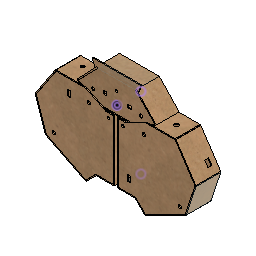
Ivrida_Digimod (Autodesk Fusion 360 design; units mm, degrees)
Autodesk Fusion 360 part; units mm, degrees
sketch "Sketch1" plane through (0, 0, 0) normal (0, 1, 0) x (1, 0, 0) in component "DigiMod"
  line L0 (0, 0) -> (120, 0)
  line L1 (120, 0) -> (160, 60)
  line L2 (160, 60) -> (140, 120)
  line L3 (140, 120) -> (60, 160)
  line L4 (60, 160) -> (40, 140)
  line L5 (40, 140) -> (-40, 140)
  line L6 (-40, 140) -> (-60, 160)
  line L7 (-60, 160) -> (-140, 120)
  line L8 (-140, 120) -> (-160, 60)
  line L9 (-160, 60) -> (-120, 0)
  line L10 (-120, 0) -> (0, 0)
  constraint coincident L0.start L10.end
  constraint horizontal L0
  constraint horizontal L5
  constraint perpendicular L4 L6
  constraint parallel L0 L10
extrude "Extrude1" add sketch "Sketch1" along normal blind 50 makes body 1 in component "DigiMod"
sketch "Sketch2" plane through (0, 0, 0) normal (0, 1, 0) x (1, 0, 0) in component "DigiMod"
  line L0 (0, 0) -> (3, 0)
  line L1 (3, 0) -> (3, 105.3915)
  line L2 (3, 105.3915) -> (3, 140)
  line L3 (3, 140) -> (-3, 140)
  line L4 (-3, 140) -> (-3, 0)
  line L5 (-3, 0) -> (0, 0)
  constraint coincident L0.start L5.end
  constraint horizontal L0
  constraint perpendicular L0 L1
  constraint perpendicular L0 L2
  constraint perpendicular L2 L3
  constraint perpendicular L3 L4
  constraint perpendicular L4 L5
extrude "Extrude2" cut sketch "Sketch2" along normal blind 48 bodies 1 in component "DigiMod"
extrude "Extrude3" add 1 faces at (27.6667, 32.6667, -140) along direction (0, 0, -1) blind 2 on bodies 1 bodies 1 in component "DigiMod"
extrude "Extrude4" cut 1 faces at (-46.6667, 16.6667, -146.6667) along direction (0.707107, 0, -0.707107) blind 2 on bodies 1 bodies 1 in component "DigiMod"
extrude "Extrude5" add 1 faces at (-86.6667, 33.3333, -146.6667) along direction (-0.447214, 0, -0.894427) blind 2 on bodies 1 bodies 1 in component "DigiMod"
extrude "Extrude6" add 1 faces at (-46.6667, 16.6667, -146.6667) along direction (0.707107, 0, -0.707107) blind 2 on bodies 1 bodies 1 in component "DigiMod"
extrude "Extrude7" add 1 faces at (-146.6667, 16.6667, -100) along direction (-0.948683, 0, -0.316228) blind 2 on bodies 1 bodies 1 in component "DigiMod"
extrude "Extrude8" add 1 faces at (-146.6667, 33.3333, -40) along direction (-0.83205, 0, 0.5547) blind 2 on bodies 1 bodies 1 in component "DigiMod"
extrude "Extrude9" add 1 faces at (-81, 32.6667, 0) along direction (0, 0, 1) blind 2 on bodies 1 bodies 1 in component "DigiMod"
extrude "Extrude10" add 1 faces at (133.3333, 33.3333, -20) along direction (0.83205, 0, 0.5547) blind 2 on bodies 1 bodies 1 in component "DigiMod"
extrude "Extrude11" add 1 faces at (153.3333, 16.6667, -80) along direction (0.948683, 0, -0.316228) blind 2 on bodies 1 bodies 1 in component "DigiMod"
extrude "Extrude12" add 1 faces at (113.3333, 16.6667, -133.3333) along direction (0.447214, 0, -0.894427) blind 2 on bodies 1 bodies 1 in component "DigiMod"
extrude "Extrude13" cut 1 faces at (53.3333, 16.6667, -153.3333) along direction (-0.707107, 0, -0.707107) blind 2 on bodies 1 bodies 1 in component "DigiMod"
extrude "Extrude14" add 1 faces at (53.3333, 16.6667, -153.3333) along direction (-0.707107, 0, -0.707107) blind 2 on bodies 1 bodies 1 in component "DigiMod"
sketch "Sketch1 (2)" plane through (0, 0, 0) normal (0, -1, 0) x (1, 0, 0)
  line L0 (-39.1716, -142) -> (-3, -142)
  line L1 (-3, -142) -> (-3, 2)
  line L2 (-3, 2) -> (-120, 2)
  line L3 (-120, 2) -> (-120, 0)
  line L4 (-120, 0) -> (-121.6641, 1.1094)
  line L5 (-121.6641, 1.1094) -> (-161.6641, -58.8906)
  line L6 (-161.6641, -58.8906) -> (-160, -60)
  line L7 (-160, -60) -> (-161.8974, -60.6325)
  line L8 (-161.8974, -60.6325) -> (-141.8974, -120.6325)
  line L9 (-141.8974, -120.6325) -> (-140, -120)
  line L10 (-140, -120) -> (-140.8944, -121.7889)
  line L11 (-140.8944, -121.7889) -> (-60.8944, -161.7889)
  line L12 (-60.8944, -161.7889) -> (-60, -160)
  line L13 (-60, -160) -> (-58.5858, -161.4142)
  line L14 (-58.5858, -161.4142) -> (-39.1716, -142)
  line L15 (-5, -140) -> (-40, -140)
  line L16 (-40, -140) -> (-60, -160)
  line L17 (-60, -160) -> (-140, -120)
  line L18 (-140, -120) -> (-160, -60)
  line L19 (-160, -60) -> (-120, 0)
  line L20 (-120, 0) -> (-75, 0)
  line L21 (-5, -140) -> (-5, -20)
  line L22 (-5, -20) -> (-40, -20)
  line L23 (-40, -20) -> (-75, 0)
  constraint perpendicular L1 L15
  constraint coincident L12.end L13.start
  constraint coincident L9.end L10.start
  constraint coincident L6.end L7.start
  constraint coincident L3.end L4.start
  constraint perpendicular L3 L20
  constraint perpendicular L15 L21
  constraint perpendicular L1 L22
extrude "Extrude15" cut sketch "Sketch1 (2)" against normal blind 48 contours L15 L16 L17 L18 L19 L20 L21 L22 L23 bodies 1 in component "DigiMod"
sketch "Sketch2 (2)" plane through (0, 0, 0) normal (0, -1, 0) x (1, 0, 0)
  line L0 (60, -160) -> (60.8944, -161.7889)
  line L1 (60.8944, -161.7889) -> (140.8944, -121.7889)
  line L2 (140.8944, -121.7889) -> (140, -120)
  line L3 (140, -120) -> (141.8974, -120.6325)
  line L4 (141.8974, -120.6325) -> (161.8974, -60.6325)
  line L5 (161.8974, -60.6325) -> (160, -60)
  line L6 (160, -60) -> (161.6641, -58.8906)
  line L7 (161.6641, -58.8906) -> (121.6641, 1.1094)
  line L8 (121.6641, 1.1094) -> (120, 0)
  line L9 (120, 0) -> (120, 2)
  line L10 (120, 2) -> (3, 2)
  line L11 (3, 2) -> (3, -142)
  line L12 (3, -142) -> (39.1716, -142)
  line L13 (39.1716, -142) -> (58.5858, -161.4142)
  line L14 (58.5858, -161.4142) -> (60, -160)
  line L15 (40, -140) -> (5, -140)
  line L16 (5, -140) -> (5, -20)
  line L17 (5, -20) -> (40, -20)
  line L18 (40, -20) -> (75, 0)
  line L19 (75, 0) -> (120, 0)
  line L20 (120, 0) -> (160, -60)
  line L21 (160, -60) -> (140, -120)
  line L22 (140, -120) -> (60, -160)
  line L23 (40, -140) -> (60, -160)
  constraint perpendicular L11 L15
  constraint perpendicular L15 L16
  constraint perpendicular L16 L17
  constraint coincident L8.end L9.start
  constraint perpendicular L9 L19
  constraint coincident L5.end L6.start
  constraint coincident L2.end L3.start
  constraint coincident L0.start L14.end
  constraint perpendicular L14 L23
extrude "Extrude16" cut sketch "Sketch2 (2)" against normal blind 48 contours L15 L16 L17 L18 L19 L20 L21 L22 L23 bodies 1 in component "DigiMod"
sketch "Sketch3" plane through (0, 0, 2) normal (0, 0, 1) x (-1, 0, 0)
  line L0 (3, 0) -> (3, -48)
  line L1 (3, -48) -> (-3, -48)
  line L2 (-3, 0) -> (-120, 0)
  line L3 (-120, 0) -> (-120, -50)
  line L4 (-120, -50) -> (120, -50)
  line L5 (120, -50) -> (120, 0)
  line L6 (120, 0) -> (3, 0)
sketch "Sketch4" plane through (0, 0, 2) normal (0, 0, 1) x (-1, 0, 0)
sketch "Sketch5" plane through (0, 0, 2) normal (0, 0, 1) x (1, 0, 0)
  line L0 (-3, 48) -> (-40, 48)
  line L1 (-40, 48) -> (-40, 0)
  line L2 (-40, 0) -> (-3, 0)
  line L3 (-3, 0) -> (-3, 48)
  point P0 (-3, 48)
  point P1 (-40, 48)
  point P2 (-40, 0)
  point P3 (-3, 0)
  constraint coincident P0 L0.start
  constraint coincident P1 L0.end
  constraint coincident P2 L1.end
  constraint coincident P3 L2.end
extrude "Extrude17" cut sketch "Sketch5" against normal blind 20 bodies 1 in component "DigiMod"
sketch "Sketch6" plane through (0, 48, 0) normal (0, -1, 0) x (1, 0, 0)
  line L0 (-3, -18) -> (-3, -142)
  line L1 (-3, -142) -> (3, -142)
  line L2 (3, 2) -> (-40, 2)
  line L3 (-40, 2) -> (-40, -18)
  line L4 (-40, -18) -> (-3, -18)
sketch "Sketch7" plane through (0, 0, 0) normal (0, -1, 0) x (1, 0, 0)
  line L0 (-3, -18) -> (-40, -18)
  line L1 (-40, -18) -> (-40, 2)
  line L2 (-40, 2) -> (-120, 2)
  line L3 (-120, 2) -> (-120, 0)
  line L4 (-120, 0) -> (-75, 0)
  line L5 (-75, 0) -> (-40, -20)
  line L6 (-40, -20) -> (-5, -20)
  line L7 (-5, -20) -> (-5, -140)
  line L8 (-5, -140) -> (-40, -140)
  line L9 (-40, -140) -> (-60, -160)
  line L10 (-60, -160) -> (-58.5858, -161.4142)
  line L11 (-58.5858, -161.4142) -> (-39.1716, -142)
  line L12 (-39.1716, -142) -> (-3, -142)
  line L13 (-3, -142) -> (-3, -18)
  line L14 (-40, 2) -> (-75, 2)
  line L15 (-75, 2) -> (-40, -18)
  constraint coincident L1.end L2.start
  constraint coincident L2 L14.end
  constraint perpendicular L1 L14
  constraint coincident L0.end L1.start
extrude "Extrude18" cut sketch "Sketch7" against normal blind 48 contours L1 L2 L14 L15 bodies 1 in component "DigiMod"
sketch "Sketch8" plane through (0, 0, 2) normal (0, 0, 1) x (-1, 0, 0)
sketch "Sketch9" plane through (0, 0, 2) normal (0, 0, 1) x (-1, 0, 0)
  point P0 (-3, 0)
sketch "Sketch10" plane through (0, 0, 2) normal (0, 0, 1) x (-1, 0, 0)
  line L0 (-3, -48) -> (-40, -48)
  line L1 (-40, -48) -> (-40, 0)
  line L2 (-40, 0) -> (-3, 0)
  line L3 (-3, 0) -> (-3, -48)
  point P0 (-3, -48)
  point P1 (-40, -48)
  point P2 (-40, 0)
  point P3 (-3, 0)
  constraint coincident P0 L0.start
  constraint coincident P1 L0.end
  constraint coincident P2 L1.end
  constraint coincident P3 L2.end
extrude "Extrude19" cut sketch "Sketch10" against normal blind 20 bodies 1 in component "DigiMod"
sketch "Sketch11" plane through (0, 0, 0) normal (0, -1, 0) x (1, 0, 0)
  line L0 (40, -18) -> (3, -18)
  line L1 (3, -18) -> (3, -142)
  line L2 (3, -142) -> (39.1716, -142)
  line L3 (39.1716, -142) -> (58.5858, -161.4142)
  line L4 (58.5858, -161.4142) -> (60, -160)
  line L5 (60, -160) -> (40, -140)
  line L6 (40, -140) -> (5, -140)
  line L7 (5, -140) -> (5, -20)
  line L8 (5, -20) -> (40, -20)
  line L9 (40, -20) -> (75, 0)
  line L10 (75, 0) -> (120, 0)
  line L11 (120, 0) -> (120, 2)
  line L12 (120, 2) -> (40, 2)
  line L13 (40, 2) -> (40, -18)
  line L14 (40, -18) -> (75, 2)
  line L15 (75, 2) -> (40, 2)
  constraint coincident L0.start L13.end
  constraint coincident L12 L14.end
  constraint coincident L12.end L13.start
extrude "Extrude20" cut sketch "Sketch11" against normal blind 48 contours L12 L13 L14 L15 bodies 1 in component "DigiMod"
delete_face "DeleteFace1" 1 faces at (15.3333, 48, -4.6667) on bodies 1 in component "DigiMod"
sketch "Sketch12" plane through (0, 48, 0) normal (0, -1, 0) x (1, 0, 0)
  line L0 (-5, -140) -> (-5, -20)
  line L1 (-5, -20) -> (-40, -20)
  line L2 (-40, -20) -> (-75, 0)
  line L3 (-75, 0) -> (-120, 0)
  line L4 (-120, 0) -> (-160, -60)
  line L5 (-160, -60) -> (-140, -120)
  line L6 (-140, -120) -> (-60, -160)
  line L7 (-60, -160) -> (-40, -140)
  line L8 (-40, -140) -> (-5, -140)
  line L9 (-120, 0) -> (-115, 0)
  line L10 (-115, 0) -> (-123.3146, -4.9719)
  constraint coincident L3.end L4.start
  constraint coincident L3 L9.end
  constraint parallel L3 L9
  constraint coincident L4 L10.end
extrude "Extrude1'" add sketch "Sketch12" along normal blind 46 separate body contours L3 L4 L9 L10 makes body 2
sketch "Sketch13" plane through (0, 48, 0) normal (0, -1, 0) x (1, 0, 0)
  line L0 (-5, -140) -> (-5, -20)
  line L1 (-5, -20) -> (-40, -20)
  line L2 (-40, -20) -> (-75, 0)
  line L3 (-75, 0) -> (-120, 0)
  line L4 (-120, 0) -> (-160, -60)
  line L5 (-160, -60) -> (-140, -120)
  line L6 (-140, -120) -> (-60, -160)
  line L7 (-60, -160) -> (-40, -140)
  line L8 (-40, -140) -> (-5, -140)
  line L9 (-75, 0) -> (-80, 0)
  line L10 (-80, 0) -> (-69.9937, -2.8607)
  constraint coincident L2.end L3.start
  constraint coincident L3 L9.end
  constraint parallel L3 L9
  constraint coincident L2 L10.end
extrude "Extrude2'" add sketch "Sketch13" along normal blind 46 separate body contours L2 L3 L9 L10 makes body 3
sketch "Sketch14" plane through (0, 48, 0) normal (0, -1, 0) x (1, 0, 0)
  line L0 (-5, -140) -> (-5, -20)
  line L1 (-5, -20) -> (-40, -20)
  line L2 (-40, -20) -> (-75, 0)
  line L3 (-75, 0) -> (-120, 0)
  line L4 (-120, 0) -> (-160, -60)
  line L5 (-160, -60) -> (-140, -120)
  line L6 (-140, -120) -> (-60, -160)
  line L7 (-60, -160) -> (-40, -140)
  line L8 (-40, -140) -> (-5, -140)
  line L9 (-5, -135) -> (-10, -140)
  constraint coincident L0 L9.start
  constraint coincident L8 L9.end
extrude "Extrude3'" add sketch "Sketch14" along normal blind 46 separate body contours L0 L8 L9 makes body 4
sketch "Sketch15" plane through (0, 48, 0) normal (0, -1, 0) x (1, 0, 0)
  line L0 (-5, -140) -> (-5, -20)
  line L1 (-5, -20) -> (-40, -20)
  line L2 (-40, -20) -> (-75, 0)
  line L3 (-75, 0) -> (-120, 0)
  line L4 (-120, 0) -> (-160, -60)
  line L5 (-160, -60) -> (-140, -120)
  line L6 (-140, -120) -> (-60, -160)
  line L7 (-60, -160) -> (-40, -140)
  line L8 (-40, -140) -> (-5, -140)
  line L9 (-60, -160) -> (-57.0566, -157.0566)
  line L10 (-65.8868, -157.0566) -> (-60, -160)
  line L11 (-65.8868, -157.0566) -> (-57.0566, -157.0566)
  constraint coincident L6.end L7.start
  constraint coincident L7 L9.end
  constraint parallel L7 L9
  constraint coincident L6 L10.start
  constraint parallel L6 L10
  constraint horizontal L11
extrude "Extrude4'" add sketch "Sketch15" along normal blind 46 separate body contours L6 L7 L9 L10 L11 makes body 5
sketch "Sketch16" plane through (0, 48, 0) normal (0, -1, 0) x (1, 0, 0)
  line L0 (-5, -140) -> (-5, -20)
  line L1 (-5, -20) -> (-40, -20)
  line L2 (-40, -20) -> (-75, 0)
  line L3 (-75, 0) -> (-120, 0)
  line L4 (-120, 0) -> (-160, -60)
  line L5 (-160, -60) -> (-140, -120)
  line L6 (-140, -120) -> (-60, -160)
  line L7 (-60, -160) -> (-40, -140)
  line L8 (-40, -140) -> (-5, -140)
  line L9 (-140, -120) -> (-141.1425, -116.5725)
  line L10 (-141.1425, -116.5725) -> (-137.5845, -116.5725)
  line L11 (-137.5845, -116.5725) -> (-137.5845, -121.2078)
  line L12 (-137.5845, -121.2078) -> (-140, -120)
  constraint coincident L5.end L6.start
  constraint coincident L5 L9.end
  constraint parallel L5 L9
  constraint horizontal L10
  constraint coincident L6 L11.end
  constraint perpendicular L10 L11
  constraint parallel L6 L12
extrude "Extrude5'" add sketch "Sketch16" along normal blind 46 separate body contours L5 L6 L9 L10 L11 L12 makes body 6
sketch "Sketch17" plane through (0, 48, 0) normal (0, -1, 0) x (1, 0, 0)
  line L0 (-5, -140) -> (-5, -20)
  line L1 (-5, -20) -> (-40, -20)
  line L2 (-40, -20) -> (-75, 0)
  line L3 (-75, 0) -> (-120, 0)
  line L4 (-120, 0) -> (-160, -60)
  line L5 (-160, -60) -> (-140, -120)
  line L6 (-140, -120) -> (-60, -160)
  line L7 (-60, -160) -> (-40, -140)
  line L8 (-40, -140) -> (-5, -140)
  line L9 (-5, -20) -> (-8.5013, -20)
  line L10 (-8.5013, -20) -> (-8.5013, -23.6443)
  line L11 (-8.5013, -23.6443) -> (-5, -23.6443)
  constraint coincident L0.end L1.start
  constraint coincident L1 L9.end
  constraint perpendicular L0 L9
  constraint perpendicular L1 L10
  constraint coincident L0 L11.end
  constraint perpendicular L0 L11
extrude "Extrude6'" add sketch "Sketch17" along normal blind 46 separate body contours L0 L1 L9 L10 L11 makes body 7
sketch "Sketch18" plane through (0, 48, 0) normal (0, -1, 0) x (1, 0, 0)
  line L0 (5, -140) -> (40, -140)
  line L1 (40, -140) -> (60, -160)
  line L2 (60, -160) -> (140, -120)
  line L3 (140, -120) -> (160, -60)
  line L4 (160, -60) -> (120, 0)
  line L5 (120, 0) -> (75, 0)
  line L6 (75, 0) -> (40, -20)
  line L7 (40, -20) -> (5, -20)
  line L8 (5, -20) -> (5, -140)
  line L9 (5, -20) -> (5, -23.6443)
  line L10 (5, -23.6443) -> (8, -23.6443)
  line L11 (8, -23.6443) -> (8, -20)
  constraint coincident L7.end L8.start
  constraint coincident L8 L9.end
  constraint perpendicular L7 L9
  constraint perpendicular L8 L10
  constraint coincident L7 L11.end
  constraint perpendicular L7 L11
extrude "Extrude7'" add sketch "Sketch18" along normal blind 46 separate body contours L7 L8 L9 L10 L11 makes body 8
sketch "Sketch19" plane through (0, 48, 0) normal (0, -1, 0) x (1, 0, 0)
  line L0 (-5, -140) -> (-5, -20)
  line L1 (-5, -20) -> (-40, -20)
  line L2 (-40, -20) -> (-75, 0)
  line L3 (-75, 0) -> (-120, 0)
  line L4 (-120, 0) -> (-160, -60)
  line L5 (-160, -60) -> (-140, -120)
  line L6 (-140, -120) -> (-60, -160)
  line L7 (-60, -160) -> (-40, -140)
  line L8 (-40, -140) -> (-5, -140)
  line L9 (-160, -60) -> (-157.8521, -56.7781)
  line L10 (-157.8521, -56.7781) -> (-158.6545, -64.0365)
  line L11 (-158.6545, -64.0365) -> (-160, -60)
  constraint coincident L4.end L5.start
  constraint coincident L4 L9.end
  constraint parallel L4 L9
  constraint coincident L5 L10.end
extrude "Extrude8'" add sketch "Sketch19" along normal blind 46 separate body contours L4 L5 L9 L10 L11 makes body 9
sketch "Sketch20" plane through (0, 48, 0) normal (0, -1, 0) x (1, 0, 0)
  line L0 (5, -140) -> (40, -140)
  line L1 (40, -140) -> (60, -160)
  line L2 (60, -160) -> (140, -120)
  line L3 (140, -120) -> (160, -60)
  line L4 (160, -60) -> (120, 0)
  line L5 (120, 0) -> (75, 0)
  line L6 (75, 0) -> (40, -20)
  line L7 (40, -20) -> (5, -20)
  line L8 (5, -20) -> (5, -140)
  line L9 (75, 0) -> (69.8639, -2.9349)
  line L10 (69.8639, -2.9349) -> (80, 0)
  line L11 (80, 0) -> (75, 0)
  constraint coincident L5.end L6.start
  constraint coincident L6 L9.end
  constraint parallel L6 L9
  constraint coincident L5 L10.end
extrude "Extrude9'" add sketch "Sketch20" along normal blind 46 separate body contours L5 L6 L9 L10 L11 makes body 10
sketch "Sketch21" plane through (0, 48, 0) normal (0, -1, 0) x (1, 0, 0)
  line L0 (5, -140) -> (40, -140)
  line L1 (40, -140) -> (60, -160)
  line L2 (60, -160) -> (140, -120)
  line L3 (140, -120) -> (160, -60)
  line L4 (160, -60) -> (120, 0)
  line L5 (120, 0) -> (75, 0)
  line L6 (75, 0) -> (40, -20)
  line L7 (40, -20) -> (5, -20)
  line L8 (5, -20) -> (5, -140)
  line L9 (120, 0) -> (115, 0)
  line L10 (115, 0) -> (122.7577, -4.1366)
  line L11 (122.7577, -4.1366) -> (120, 0)
  constraint coincident L4.end L5.start
  constraint coincident L5 L9.end
  constraint parallel L5 L9
  constraint coincident L4 L10.end
extrude "Extrude10'" add sketch "Sketch21" along normal blind 46 separate body contours L4 L5 L9 L10 L11 makes body 11
sketch "Sketch22" plane through (0, 48, 0) normal (0, -1, 0) x (1, 0, 0)
  line L0 (5, -140) -> (40, -140)
  line L1 (40, -140) -> (60, -160)
  line L2 (60, -160) -> (140, -120)
  line L3 (140, -120) -> (160, -60)
  line L4 (160, -60) -> (120, 0)
  line L5 (120, 0) -> (75, 0)
  line L6 (75, 0) -> (40, -20)
  line L7 (40, -20) -> (5, -20)
  line L8 (5, -20) -> (5, -140)
  line L9 (160, -60) -> (156.4985, -54.7478)
  line L10 (156.4985, -54.7478) -> (154.7478, -60)
  line L11 (154.7478, -60) -> (158.9277, -63.2168)
  constraint coincident L3.end L4.start
  constraint coincident L4 L9.end
  constraint parallel L3 L10
  constraint coincident L3 L11.end
extrude "Extrude11'" add sketch "Sketch22" along normal blind 46 separate body contours L3 L4 L9 L10 L11 makes body 12
sketch "Sketch23" plane through (0, 48, 0) normal (0, -1, 0) x (1, 0, 0)
  line L0 (5, -140) -> (40, -140)
  line L1 (40, -140) -> (60, -160)
  line L2 (60, -160) -> (140, -120)
  line L3 (140, -120) -> (160, -60)
  line L4 (160, -60) -> (120, 0)
  line L5 (120, 0) -> (75, 0)
  line L6 (75, 0) -> (40, -20)
  line L7 (40, -20) -> (5, -20)
  line L8 (5, -20) -> (5, -140)
  line L9 (140, -120) -> (135.3388, -122.3306)
  line L10 (135.3388, -122.3306) -> (135.3388, -117)
  line L11 (135.3388, -117) -> (141, -117)
  constraint coincident L2.end L3.start
  constraint coincident L2 L9.end
  constraint parallel L2 L9
  constraint vertical L10
  constraint coincident L3 L11.end
  constraint perpendicular L10 L11
extrude "Extrude12'" add sketch "Sketch23" along normal blind 46 separate body contours L2 L3 L9 L10 L11 makes body 13
sketch "Sketch24" plane through (0, 48, 0) normal (0, -1, 0) x (1, 0, 0)
  line L0 (5, -140) -> (40, -140)
  line L1 (40, -140) -> (60, -160)
  line L2 (60, -160) -> (140, -120)
  line L3 (140, -120) -> (160, -60)
  line L4 (160, -60) -> (120, 0)
  line L5 (120, 0) -> (75, 0)
  line L6 (75, 0) -> (40, -20)
  line L7 (40, -20) -> (5, -20)
  line L8 (5, -20) -> (5, -140)
  line L9 (60, -160) -> (65.1873, -157.4063)
  line L10 (57, -157) -> (60, -160)
  line L11 (57, -157) -> (65.1873, -157.4063)
  constraint coincident L1.end L2.start
  constraint coincident L2 L9.end
  constraint parallel L2 L9
  constraint coincident L1 L10.start
extrude "Extrude13'" add sketch "Sketch24" along normal blind 46 separate body contours L1 L2 L9 L10 L11 makes body 14
sketch "Sketch25" plane through (0, 48, 0) normal (0, -1, 0) x (1, 0, 0)
  line L0 (5, -140) -> (40, -140)
  line L1 (40, -140) -> (60, -160)
  line L2 (60, -160) -> (140, -120)
  line L3 (140, -120) -> (160, -60)
  line L4 (160, -60) -> (120, 0)
  line L5 (120, 0) -> (75, 0)
  line L6 (75, 0) -> (40, -20)
  line L7 (40, -20) -> (5, -20)
  line L8 (5, -20) -> (5, -140)
  line L9 (5, -140) -> (10, -140)
  line L10 (10, -140) -> (5, -135)
  constraint coincident L0.start L8.end
  constraint coincident L0 L9.end
  constraint perpendicular L8 L9
  constraint coincident L8 L10.end
extrude "Extrude14'" add sketch "Sketch25" along normal blind 46 separate body contours L0 L8 L9 L10 makes body 15
hole "Hole1" at (96.9323, 25.2831, 2) direction (0, 0, -1) diameter 8.7 depth 60 tip angle 118 bodies 1 in component "DigiMod"
hole "Hole2" at (-98.9314, 32.8957, 2) direction (0, 0, -1) diameter 7.4 depth 60 tip angle 118 bodies 1 in component "DigiMod"
hole "Hole3" at (-21.5, 24, -18) direction (0, 0, -1) diameter 8.7 depth 60 tip angle 118 bodies 1 in component "DigiMod"
sketch "Sketch26" plane through (51.4142, 0, -51.4142) normal (0.707107, 0, -0.707107) x (0, 1, 0)
  line L0 (50, -128.1077) -> (0, -128.1077)
  line L1 (0, -128.1077) -> (0, -155.5635)
  line L2 (0, -155.5635) -> (50, -155.5635)
  line L3 (50, -155.5635) -> (50, -128.1077)
  line L4 (47, -145) -> (47, -133)
  line L5 (47, -133) -> (37, -133)
  line L6 (37, -133) -> (37, -145)
  line L7 (37, -145) -> (47, -145)
  constraint parallel L3 L4
  constraint perpendicular L3 L5
  constraint perpendicular L5 L6
  constraint perpendicular L4 L7
extrude "Extrude21" cut sketch "Sketch26" against normal blind 3 contours L4 L5 L6 L7 bodies 1 in component "DigiMod"
sketch "Sketch27" plane through (163.8974, 0, -54.6325) normal (0.948683, 0, -0.316228) x (0, 1, 0)
  line L0 (0, -6.3246) -> (0, -69.5701)
  line L1 (0, -69.5701) -> (50, -69.5701)
  line L2 (50, -69.5701) -> (50, -6.3246)
  line L3 (50, -6.3246) -> (0, -6.3246)
sketch "Sketch28" plane through (84.741, 0, 56.494) normal (0.83205, 0, 0.5547) x (0, 1, 0)
  line L0 (0, -66.564) -> (0, -138.675)
  line L1 (0, -138.675) -> (50, -138.675)
  line L2 (50, -138.675) -> (50, -66.564)
  line L3 (50, -66.564) -> (0, -66.564)
  line L4 (40, -125) -> (40, -113)
  line L5 (40, -113) -> (32, -113)
  line L6 (32, -113) -> (32, -125)
  line L7 (32, -125) -> (40, -125)
  constraint vertical L4
  constraint perpendicular L4 L5
  constraint perpendicular L5 L6
  constraint perpendicular L4 L7
extrude "Extrude22" cut sketch "Sketch28" against normal blind 5 contours L4 L5 L6 L7 bodies 1 in component "DigiMod"
sketch "Sketch29" plane through (5, 0, 0) normal (1, 0, 0) x (0, 1, 0)
  line L0 (0, -20) -> (0, -140)
  line L1 (0, -140) -> (48, -140)
  line L2 (48, -140) -> (48, -20)
  line L3 (48, -20) -> (0, -20)
  line L4 (48, -29.8881) -> (28, -29.8881)
  line L5 (28, -29.8881) -> (28, -62)
  line L6 (28, -62) -> (48, -62)
  line L7 (28, -62) -> (28, -29.8881)
  line L8 (48, -29.8881) -> (48, -62)
  constraint coincident L2 L4.start
  constraint perpendicular L2 L4
  constraint perpendicular L4 L5
  constraint coincident L2 L6.end
  constraint perpendicular L2 L6
extrude "Extrude23" cut sketch "Sketch29" against normal blind 60 contours L2 L4 L5 L6 L7 L8 bodies 1 in component "DigiMod"
sketch "Sketch7 (2)" plane through (0, 0, 0) normal (0, -1, 0) x (1, 0, 0) in component "DigiMod"
  line L0 (5, -20) -> (40, -20)
  line L1 (40, -20) -> (75, 0)
  line L2 (75, 0) -> (75, 2)
  line L3 (75, 2) -> (40, -18)
  line L4 (40, -18) -> (3, -18)
  line L5 (40, -18) -> (5, -18)
  line L6 (5, -18) -> (5, -20)
  point P0 (5, -20)
  point P1 (40, -20)
  point P2 (75, 0)
  point P3 (75, 2)
  point P4 (40, -18)
  constraint coincident P0 L0.start
  constraint coincident P1 L0.end
  constraint coincident P2 L1.end
  constraint coincident P3 L2.end
  constraint coincident P4 L3.end
  constraint coincident L4 L5.end
  constraint parallel L0 L5
  constraint perpendicular L0 L6
sketch "Sketch8 (2)" plane through (0, 48, 0) normal (0, -1, 0) x (1, 0, 0) in component "DigiMod"
  line L0 (-3, -62) -> (-3, -142)
  line L1 (-3, -142) -> (3, -142)
  line L2 (3, -142) -> (3, -62)
  line L3 (3, -62) -> (5, -62)
  line L4 (5, -62) -> (5, -140)
  line L5 (5, -140) -> (40, -140)
  line L6 (40, -140) -> (60, -160)
  line L7 (60, -160) -> (140, -120)
  line L8 (140, -120) -> (160, -60)
  line L9 (160, -60) -> (120, 0)
  line L10 (120, 0) -> (75, 0)
  line L11 (75, 0) -> (40, -20)
  line L12 (40, -20) -> (5, -20)
  line L13 (5, -20) -> (5, -29.8881)
  line L14 (5, -29.8881) -> (3, -29.8881)
  line L15 (3, -29.8881) -> (3, -18)
  line L16 (3, -18) -> (40, -18)
  line L17 (40, -18) -> (75, 2)
  line L18 (-75, 2) -> (-40, -18)
  line L19 (-40, -18) -> (-3, -18)
  line L20 (-3, -18) -> (-3, -29.8881)
  line L21 (-3, -29.8881) -> (-5, -29.8881)
  line L22 (-5, -29.8881) -> (-5, -20)
  line L23 (-5, -20) -> (-40, -20)
  line L24 (-40, -20) -> (-75, 0)
  line L25 (-75, 0) -> (-120, 0)
  line L26 (-120, 0) -> (-160, -60)
  line L27 (-160, -60) -> (-140, -120)
  line L28 (-140, -120) -> (-60, -160)
  line L29 (-60, -160) -> (-40, -140)
  line L30 (-40, -140) -> (-5, -140)
  line L31 (-5, -140) -> (-5, -62)
  line L32 (-5, -62) -> (-3, -62)
  line L33 (-40, -18) -> (40, -18)
  line L34 (40, -18) -> (80.0335, 4.8763)
  line L35 (80.0335, 4.8763) -> (40, 47)
  line L36 (40, 47) -> (-40, 47)
  line L37 (-40, 47) -> (40, 47)
  line L38 (40, 47) -> (80.0335, 4.8763)
  line L39 (-40, 47) -> (-79.9003, 4.8763)
  line L40 (-79.9003, 4.8763) -> (-40, 47)
  line L41 (-79.9003, 4.8763) -> (-40, -18)
  constraint coincident L18.end L19.start
  constraint coincident L16.end L17.start
  constraint parallel L17 L34
  constraint parallel L33 L36
  constraint parallel L36 L37
  constraint parallel L35 L38
  constraint parallel L39 L40
extrude "Extrude27" cut sketch "Sketch7 (2)" against normal blind 2 bodies 1 in component "DigiMod"
sketch "Sketch9 (2)" plane through (0, 48, 0) normal (0, -1, 0) x (1, 0, 0) in component "DigiMod"
  line L0 (-5, -20, 48) -> (-40, -20, 48)
  line L1 (-40, -20, 48) -> (-75, 0, 48)
  line L2 (-75, 0, 48) -> (-75, 2, 48)
  line L3 (-75, 2, 48) -> (-40, -18, 48)
  line L4 (-3, -18, 48) -> (-40, -18, 48)
  line L5 (-40, -18, 48) -> (-5.0165, -18, 48)
  line L6 (-5.0165, -18, 48) -> (-5, -20, 48)
  line L7 (-5.0165, -18, 48) -> (-40, -18, 48)
  point P0 (-5, -20)
  point P1 (-40, -20)
  point P2 (-75, 0)
  point P3 (-75, 2)
  point P4 (-40, -18)
  point P5 (-40, -18)
  constraint coincident P5 P4
extrude "Extrude28" cut sketch "Sketch9 (2)" against normal blind 2 contours L0 L1 L2 L3 L4 L5 L6 L7 in plane through (0, 0, 0) normal (0, -1, 0) bodies 1 in component "DigiMod"
ref_plane "WorkPlane1" through (0, 0, 0) normal (0, 1, 0) x (0, 0, 1) in component "Tapas DigiMod"
sketch "Sketch1 (3)" plane through (0, 0, 0) normal (0, -1, 0) x (1, 0, 0) in component "Tapas DigiMod"
  line L0 (75, 2) -> (75, 0)
  line L1 (75, 0) -> (120, 0)
  line L2 (120, 0) -> (120, 2)
  line L3 (120, 2) -> (75, 2)
  line L4 (75, 0) -> (120, 0)
  line L5 (120, 0) -> (160, -60)
  line L6 (160, -60) -> (140, -120)
  line L7 (140, -120) -> (60, -160)
  line L8 (60, -160) -> (40, -140)
  line L9 (40, -140) -> (5, -140)
  line L10 (5, -20) -> (5, -140)
  line L11 (5, -20) -> (20, -20)
  line L12 (20, -20) -> (5, -20)
  line L13 (5, -20) -> (20, -20)
  line L14 (60, 0) -> (20, -20)
  line L15 (60, 0) -> (75, 0)
  line L16 (75, 0) -> (60, 0)
  line L17 (60, 0) -> (20, -20)
  line L18 (20, -20) -> (60, 0)
  line L19 (20, -20) -> (60, 0)
  point P0 (160, -60)
  point P1 (140, -120)
  point P2 (60, -160)
  point P3 (40, -140)
  point P4 (5, -140)
  constraint coincident L0.end L1.start
  constraint coincident L1.end L2.start
  constraint coincident P0 L5.end
  constraint coincident P1 L6.end
  constraint coincident P2 L7.end
  constraint coincident P3 L8.end
  constraint coincident P4 L9.end
  constraint perpendicular L9 L10
  constraint perpendicular L10 L11
  constraint parallel L1 L15
  constraint parallel L14 L17
  constraint parallel L17 L18
  constraint parallel L18 L19
sketch "Sketch2 (3)" plane through (0, 0, 0) normal (0, -1, 0) x (1, 0, 0) in component "Tapas DigiMod"
extrude "Extrude1''" add sketch "Sketch1 (3)" against normal blind 2 separate body contours L1 L4 L5 L6 L7 L8 L9 L10 L11 L12 L13 L14 L15 L16 L17 L18 L19 makes body 16 in component "Tapas DigiMod"
copy_body "CopyPasteBodies1" bodies 16 makes body 17 in component "Tapas DigiMod"
move_body "Move1" bodies 17 to x (-1, 0, 0) y (0, -1, 0) z (0, 0, 1) at (0.3228, 0, 0.2253) in component "Tapas DigiMod"
move_body "Move2" bodies 17 to x (1, 0, 0) y (0, 1, 0) z (0, 0, 1) at (0, 2.0275, -0.2253) in component "Tapas DigiMod"
hole "Hole1'" at (-14.1817, 0.0275, -28.8279) direction (0, 1, 0) diameter 5 depth 10 tip angle 118 bodies 17 in component "Tapas DigiMod"
hole "Hole2'" at (14.6828, 0, -28.2508) direction (0, 1, 0) diameter 6 depth 10 tip angle 118 bodies 16 in component "Tapas DigiMod"
hole "Hole3'" at (-124.3556, 0.0275, -109.5658) direction (0, 1, 0) diameter 7 depth 10 tip angle 118 bodies 17 in component "Tapas DigiMod"
hole "Hole4" at (129.3585, 0, -111.925) direction (0, 1, 0) diameter 7 depth 10 tip angle 118 bodies 16 in component "Tapas DigiMod"
hole "Hole5" at (57.1125, 0, -22.0173) direction (0, 1, 0) diameter 7 depth 10 tip angle 118 bodies 16 in component "Tapas DigiMod"
hole "Hole6" at (-53.8278, 0.0275, -21.8662) direction (0, 1, 0) diameter 7 depth 10 tip angle 118 bodies 17 in component "Tapas DigiMod"
sketch "Sketch3 (2)" plane through (0, 0.0275, 0) normal (0, -1, 0) x (1, 0, 0) in component "Tapas DigiMod"
  circle A0 centre (-53.8278, -21.8662) radius 3.5
  circle A1 centre (-124.3556, -109.5658) radius 3.5
  circle A2 centre (-14.1817, -28.8279) radius 2.5
  line L0 (-4.6772, -140) -> (-4.6772, -20)
  line L1 (-4.6772, -20) -> (-19.6772, -20)
  line L2 (-19.6772, -20) -> (-59.6772, 0)
  line L3 (-59.6772, 0) -> (-119.6772, 0)
  line L4 (-119.6772, 0) -> (-159.6772, -60)
  line L5 (-159.6772, -60) -> (-139.6772, -120)
  line L6 (-139.6772, -120) -> (-59.6772, -160)
  line L7 (-59.6772, -160) -> (-39.6772, -140)
  line L8 (-39.6772, -140) -> (-4.6772, -140)
  line L9 (-90, -20) -> (-90, -32)
  line L10 (-90, -32) -> (-96, -32)
  line L11 (-96, -32) -> (-96, -20)
  line L12 (-96, -20) -> (-90, -20)
  constraint vertical L9
  constraint perpendicular L9 L10
  constraint perpendicular L10 L11
  constraint perpendicular L9 L12
extrude "Extrude2''" cut sketch "Sketch3 (2)" against normal blind 5 contours L9 L10 L11 L12 bodies 17 in component "Tapas DigiMod"
sketch "Sketch4 (2)" plane through (0, 0, 0) normal (0, -1, 0) x (1, 0, 0) in component "Tapas DigiMod"
  circle A0 centre (57.1125, -22.0173) radius 3.5
  circle A1 centre (129.3585, -111.925) radius 3.5
  circle A2 centre (14.6828, -28.2508) radius 3
  line L0 (5, -20) -> (5, -140)
  line L1 (5, -140) -> (40, -140)
  line L2 (40, -140) -> (60, -160)
  line L3 (60, -160) -> (140, -120)
  line L4 (140, -120) -> (160, -60)
  line L5 (160, -60) -> (120, 0)
  line L6 (120, 0) -> (60, 0)
  line L7 (60, 0) -> (20, -20)
  line L8 (20, -20) -> (5, -20)
  line L9 (30, -120) -> (30, -108)
  line L10 (30, -108) -> (24, -108)
  line L11 (24, -108) -> (24, -120)
  line L12 (24, -120) -> (30, -120)
  constraint vertical L9
  constraint perpendicular L9 L10
  constraint perpendicular L10 L11
  constraint perpendicular L9 L12
extrude "Extrude3''" cut sketch "Sketch4 (2)" against normal blind 5 contours L9 L10 L11 L12 bodies 16 in component "Tapas DigiMod"
ref_plane "WorkPlane1" through (0, 0, 0) normal (0, 1, 0) x (0, 0, 1) in component "Tapas DigiMod (1)"
sketch "Sketch1 (4)" plane through (0, 0, 0) normal (0, -1, 0) x (1, 0, 0) in component "Tapas DigiMod (1)"
  line L0 (75, 2) -> (75, 0)
  line L1 (75, 0) -> (120, 0)
  line L2 (120, 0) -> (120, 2)
  line L3 (120, 2) -> (75, 2)
  line L4 (75, 0) -> (120, 0)
  line L5 (120, 0) -> (160, -60)
  line L6 (160, -60) -> (140, -120)
  line L7 (140, -120) -> (60, -160)
  line L8 (60, -160) -> (40, -140)
  line L9 (40, -140) -> (5, -140)
  line L10 (5, -20) -> (5, -140)
  line L11 (5, -20) -> (20, -20)
  line L12 (20, -20) -> (5, -20)
  line L13 (5, -20) -> (20, -20)
  line L14 (60, 0) -> (20, -20)
  line L15 (60, 0) -> (75, 0)
  line L16 (75, 0) -> (60, 0)
  line L17 (60, 0) -> (20, -20)
  line L18 (20, -20) -> (60, 0)
  line L19 (20, -20) -> (60, 0)
  point P0 (160, -60)
  point P1 (140, -120)
  point P2 (60, -160)
  point P3 (40, -140)
  point P4 (5, -140)
  constraint coincident L0.end L1.start
  constraint coincident L1.end L2.start
  constraint coincident P0 L5.end
  constraint coincident P1 L6.end
  constraint coincident P2 L7.end
  constraint coincident P3 L8.end
  constraint coincident P4 L9.end
  constraint perpendicular L9 L10
  constraint perpendicular L10 L11
  constraint parallel L1 L15
  constraint parallel L14 L17
  constraint parallel L17 L18
  constraint parallel L18 L19
sketch "Sketch2 (4)" plane through (0, 0, 0) normal (0, -1, 0) x (1, 0, 0) in component "Tapas DigiMod (1)"
extrude "Extrude1'''" add sketch "Sketch1 (4)" against normal blind 2 separate body contours L1 L4 L5 L6 L7 L8 L9 L10 L11 L12 L13 L14 L15 L16 L17 L18 L19 makes body 18 in component "Tapas DigiMod (1)"
copy_body "CopyPasteBodies1'" bodies 18 makes body 19 in component "Tapas DigiMod (1)"
move_body "Move1'" bodies 19 to x (-1, 0, 0) y (0, -1, 0) z (0, 0, 1) at (0.3228, 0, 0.2253) in component "Tapas DigiMod (1)"
move_body "Move2'" bodies 19 to x (1, 0, 0) y (0, 1, 0) z (0, 0, 1) at (0, 2.0275, -0.2253) in component "Tapas DigiMod (1)"
hole "Hole1''" at (-14.1817, 0.0275, -28.8279) direction (0, 1, 0) diameter 5 depth 10 tip angle 118 bodies 19 in component "Tapas DigiMod (1)"
hole "Hole2''" at (14.6828, 0, -28.2508) direction (0, 1, 0) diameter 6 depth 10 tip angle 118 bodies 18 in component "Tapas DigiMod (1)"
hole "Hole3''" at (-124.3556, 0.0275, -109.5658) direction (0, 1, 0) diameter 7 depth 10 tip angle 118 bodies 19 in component "Tapas DigiMod (1)"
hole "Hole4'" at (129.3585, 0, -111.925) direction (0, 1, 0) diameter 7 depth 10 tip angle 118 bodies 18 in component "Tapas DigiMod (1)"
hole "Hole5'" at (57.1125, 0, -22.0173) direction (0, 1, 0) diameter 7 depth 10 tip angle 118 bodies 18 in component "Tapas DigiMod (1)"
hole "Hole6'" at (-53.8278, 0.0275, -21.8662) direction (0, 1, 0) diameter 7 depth 10 tip angle 118 bodies 19 in component "Tapas DigiMod (1)"
sketch "Sketch3 (3)" plane through (0, 0.0275, 0) normal (0, -1, 0) x (1, 0, 0) in component "Tapas DigiMod (1)"
  circle A0 centre (-53.8278, -21.8662) radius 3.5
  circle A1 centre (-124.3556, -109.5658) radius 3.5
  circle A2 centre (-14.1817, -28.8279) radius 2.5
  line L0 (-4.6772, -140) -> (-4.6772, -20)
  line L1 (-4.6772, -20) -> (-19.6772, -20)
  line L2 (-19.6772, -20) -> (-59.6772, 0)
  line L3 (-59.6772, 0) -> (-119.6772, 0)
  line L4 (-119.6772, 0) -> (-159.6772, -60)
  line L5 (-159.6772, -60) -> (-139.6772, -120)
  line L6 (-139.6772, -120) -> (-59.6772, -160)
  line L7 (-59.6772, -160) -> (-39.6772, -140)
  line L8 (-39.6772, -140) -> (-4.6772, -140)
  line L9 (-90, -20) -> (-90, -32)
  line L10 (-90, -32) -> (-96, -32)
  line L11 (-96, -32) -> (-96, -20)
  line L12 (-96, -20) -> (-90, -20)
  constraint vertical L9
  constraint perpendicular L9 L10
  constraint perpendicular L10 L11
  constraint perpendicular L9 L12
extrude "Extrude2'''" cut sketch "Sketch3 (3)" against normal blind 5 contours L9 L10 L11 L12 bodies 19 in component "Tapas DigiMod (1)"
sketch "Sketch4 (3)" plane through (0, 0, 0) normal (0, -1, 0) x (1, 0, 0) in component "Tapas DigiMod (1)"
  circle A0 centre (57.1125, -22.0173) radius 3.5
  circle A1 centre (129.3585, -111.925) radius 3.5
  circle A2 centre (14.6828, -28.2508) radius 3
  line L0 (5, -20) -> (5, -140)
  line L1 (5, -140) -> (40, -140)
  line L2 (40, -140) -> (60, -160)
  line L3 (60, -160) -> (140, -120)
  line L4 (140, -120) -> (160, -60)
  line L5 (160, -60) -> (120, 0)
  line L6 (120, 0) -> (60, 0)
  line L7 (60, 0) -> (20, -20)
  line L8 (20, -20) -> (5, -20)
  line L9 (30, -120) -> (30, -108)
  line L10 (30, -108) -> (24, -108)
  line L11 (24, -108) -> (24, -120)
  line L12 (24, -120) -> (30, -120)
  constraint vertical L9
  constraint perpendicular L9 L10
  constraint perpendicular L10 L11
  constraint perpendicular L9 L12
extrude "Extrude3'''" cut sketch "Sketch4 (3)" against normal blind 5 contours L9 L10 L11 L12 bodies 18 in component "Tapas DigiMod (1)"
ref_plane "WorkPlane1" through (0, 0, 0) normal (0, 1, 0) x (0, 0, 1) in component "NebuloSubmod"
extrude "Extrude1''''" add sketch "Sketch8 (2)" along normal blind 46 separate body contours L16 L17 L19 L33 L34 L35 L36 L37 L38 L39 L40 L41 makes body 20 in component "NebuloSubmod"
sketch "Sketch1 (5)" plane through (0, 2, 0) normal (0, -1, 0) x (1, 0, 0) in component "NebuloSubmod"
  line L0 (-40, 47) -> (-79.9003, 4.8763)
  line L1 (-79.9003, 4.8763) -> (-40, -18)
  line L2 (-40, -18) -> (40, -18)
  line L3 (40, -18) -> (80.0335, 4.8763)
  line L4 (80.0335, 4.8763) -> (40, 47)
  line L5 (40, 47) -> (-40, 47)
  line L6 (38, -16) -> (77, 5)
  line L7 (77, 5) -> (38, 45)
  line L8 (38, 45) -> (-38, 45)
  line L9 (38, -16) -> (-38, -16)
  line L10 (-38, -16) -> (-77, 5)
  line L11 (-77, 5) -> (-38, 45)
  constraint parallel L5 L8
  constraint parallel L2 L9
extrude "Extrude2''''" cut sketch "Sketch1 (5)" against normal blind 44 contours L6 L7 L8 L9 L10 L11 bodies 20 in component "NebuloSubmod"
sketch "Sketch2 (5)" plane through (0, 46, 0) normal (0, -1, 0) x (1, 0, 0) in component "NebuloSubmod"
  line L0 (38, -16) -> (77, 5)
  line L1 (77, 5) -> (38, 45)
  line L2 (38, 45) -> (-38, 45)
  line L3 (-38, 45) -> (-77, 5)
  line L4 (-77, 5) -> (-38, -16)
  line L5 (-38, -16) -> (38, -16)
  line L6 (-72.9911, 9.1117) -> (-72.9911, 2.8414)
  constraint coincident L3 L6.start
  constraint coincident L4 L6.end
  constraint vertical L6
extrude "Extrude3''''" add sketch "Sketch2 (5)" along normal blind 42 contours L3 L4 L6 bodies 20 in component "NebuloSubmod"
sketch "Sketch3 (4)" plane through (0, 46, 0) normal (0, -1, 0) x (1, 0, 0) in component "NebuloSubmod"
  line L0 (-72.9911, 9.1117) -> (-72.9911, 2.8414)
  line L1 (-72.9911, 2.8414) -> (-38, -16)
  line L2 (-38, -16) -> (38, -16)
  line L3 (38, -16) -> (77, 5)
  line L4 (77, 5) -> (38, 45)
  line L5 (38, 45) -> (-38, 45)
  line L6 (-38, 45) -> (-72.9911, 9.1117)
  line L7 (73.0586, 9.0424) -> (73.0586, 2.8777)
  constraint coincident L4 L7.start
  constraint coincident L3 L7.end
  constraint vertical L7
extrude "Extrude4''" add sketch "Sketch3 (4)" along normal blind 42 contours L3 L4 L7 bodies 20 in component "NebuloSubmod"
sketch "Sketch4 (4)" plane through (0, 0, 45) normal (0, 0, -1) x (1, 0, 0) in component "NebuloSubmod"
  line L0 (38, -2) -> (-38, -2)
  line L1 (-38, -2) -> (-38, -46)
  line L2 (-38, -46) -> (38, -46)
  line L3 (38, -46) -> (38, -2)
sketch "Sketch5 (2)" plane through (0, 2, 0) normal (0, -1, 0) x (1, 0, 0) in component "NebuloSubmod"
  line L0 (38, 45) -> (77, 5)
  line L1 (77, 5) -> (38, -16)
  line L2 (38, -16) -> (-38, -16)
  line L3 (-38, -16) -> (-77, 5)
  line L4 (-77, 5) -> (-38, 45)
  line L5 (-38, 45) -> (38, 45)
  line L6 (-40, 47) -> (-79.9003, 4.8763)
  line L7 (-79.9003, 4.8763) -> (-40, -18)
  line L8 (-40, -18) -> (40, -18)
  line L9 (40, -18) -> (80.0335, 4.8763)
  line L10 (80.0335, 4.8763) -> (40, 47)
  line L11 (40, 47) -> (-40, 47)
  line L12 (-38, 45) -> (-40, 47)
  line L13 (40, 47) -> (38, 45)
  constraint coincident L4.end L5.start
  constraint coincident L6.start L11.end
  constraint coincident L10.end L11.start
  constraint coincident L0.start L5.end
extrude "Extrude5''" cut sketch "Sketch5 (2)" against normal blind 6 contours L5 L11 L12 L13 bodies 20 in component "NebuloSubmod"
sketch "Sketch6 (2)" plane through (0, 0, 45) normal (0, 0, -1) x (1, 0, 0) in component "NebuloSubmod"
  line L0 (34.9057, -4.0075, 61) -> (-35, -4.0075, 61)
  line L1 (-35, -4.0075, 61) -> (-35, -7, 61)
  line L2 (-35, -7, 61) -> (34.9057, -7, 61)
  line L3 (34.9057, -7, 61) -> (34.9057, -4.0075, 61)
extrude "Extrude6''" add sketch "Sketch6 (2)" against normal blind 2 contours L0 L1 L2 L3 in plane through (0, 0, -16) normal (0, 0, -1) bodies 20 in component "NebuloSubmod"
sketch "Sketch7 (3)" plane through (0, 0, 45) normal (0, 0, -1) x (1, 0, 0) in component "NebuloSubmod"
  line L0 (38, -8) -> (-38, -8)
  line L1 (-38, -8) -> (-38, -46)
  line L2 (-38, -46) -> (38, -46)
  line L3 (38, -46) -> (38, -8)
sketch "Sketch8 (3)" plane through (41.9737, 0, 40.9244) normal (-0.716, 0, -0.6981) x (0, -1, 0) in component "NebuloSubmod"
  line L0 (-4, -44.5279) -> (-4, -50.1737)
  line L1 (-4, -50.1737) -> (-2, -50.1737)
  line L2 (-2, -50.1737) -> (-2, 5.6922)
  line L3 (-2, 5.6922) -> (-8, 5.6922)
  line L4 (-8, 5.6922) -> (-46, 5.6922)
  line L5 (-46, 5.6922) -> (-46, -44.5279)
  line L6 (-46, -44.5279) -> (-4, -44.5279)
  line L7 (-5, 1.7226) -> (-14, 1.7226)
  line L8 (-14, 1.7226) -> (-14, 5)
  line L9 (-14, 5) -> (-5, 5)
  line L10 (-5, 5) -> (-5, 1.7226)
  constraint horizontal L7
  constraint vertical L8
  constraint horizontal L9
  constraint vertical L10
extrude "Extrude7''" add sketch "Sketch8 (3)" along normal blind 2 contours L7 L8 L9 L10 bodies 20 in component "NebuloSubmod"
sketch "Sketch9 (3)" plane through (-41.9737, 0, 40.9244) normal (0.716, 0, -0.6981) x (0, 1, 0) in component "NebuloSubmod"
  line L0 (4, -50.1737) -> (4, -44.4311)
  line L1 (4, -44.4311) -> (46, -44.4311)
  line L2 (46, -44.4311) -> (46, 5.6922)
  line L3 (46, 5.6922) -> (8, 5.6922)
  line L4 (8, 5.6922) -> (2, 5.6922)
  line L5 (2, 5.6922) -> (2, -50.1737)
  line L6 (2, -50.1737) -> (4, -50.1737)
  line L7 (15, 4) -> (5, 4)
  line L8 (5, 4) -> (5, 1)
  line L9 (5, 1) -> (15, 1)
  line L10 (15, 1) -> (15, 4)
  constraint horizontal L7
  constraint vertical L8
  constraint horizontal L9
  constraint vertical L10
extrude "Extrude8''" add sketch "Sketch9 (3)" along normal blind 2 contours L7 L8 L9 L10 bodies 20 in component "NebuloSubmod"
hole "Hole1'''" at (-22.5428, 25.1997, -16) direction (0, 0, -1) diameter 5 depth 2 tip angle 118 bodies 20 in component "NebuloSubmod"
ref_plane "WorkPlane1" through (0, 0, 0) normal (0, 1, 0) x (0, 0, 1) in component "Tapa Nebulo"
sketch "Sketch1 (6)" plane through (0, 0, 0) normal (0, 1, 0) x (1, 0, 0) in component "Tapa Nebulo"
  line L0 (-38, -45, 2) -> (-77, -5, 2)
  line L1 (-77, -5, 2) -> (-38, 16, 2)
  line L2 (-38, 16, 2) -> (38, 16, 2)
  line L3 (38, 16, 2) -> (77, -5, 2)
  line L4 (77, -5, 2) -> (38, -45, 2)
  line L5 (38, -45, 2) -> (-38, -45, 2)
  line L6 (38, -45, 2) -> (40, -47, 2)
  line L7 (40, -47, 2) -> (43.5784, -43.2525, 2)
  line L8 (43.5784, -43.2525, 2) -> (48.5784, -58.2525, 2)
  line L9 (48.5784, -58.2525, 2) -> (-49.7939, -58.2525, 2)
  line L10 (-49.7939, -58.2525, 2) -> (-43.5815, -43.2263, 2)
  line L11 (-43.5815, -43.2263, 2) -> (-39.9963, -46.9968, 2)
  line L12 (-39.9963, -46.9968, 2) -> (-37.9795, -45, 2)
  point P0 (-38, -45)
  point P1 (38, 16)
  point P2 (77, -5)
  point P3 (38, -45)
extrude "Extrude1'''''" add sketch "Sketch1 (6)" along normal blind 2 separate body contours L0 L1 L2 L3 L4 L5 | L5 L6 L7 L8 L9 L10 L11 L12 in plane through (0, 2, 0) normal (0, 1, 0) makes body 21 in component "Tapa Nebulo"
hole "Hole1''''" at (-0.0751, 2, 0.0768) direction (0, 1, 0) diameter 6.7 depth 25 tip angle 118 bodies 21 in component "Tapa Nebulo"
hole "Hole2'''" at (48.4749, 2, 5.0884) direction (0, 1, 0) diameter 6.7 depth 25 tip angle 118 bodies 21 in component "Tapa Nebulo"
hole "Hole3'''" at (-47.3721, 2, 4.6708) direction (0, 1, 0) diameter 6.7 depth 25 tip angle 118 bodies 21 in component "Tapa Nebulo"
hole "Hole4''" at (-0.075, 2, 24.8216) direction (0, 1, 0) diameter 5 depth 25 tip angle 118 bodies 21 in component "Tapa Nebulo"
sketch "Sketch2 (6)" plane through (0, 2, 0) normal (0, -1, 0) x (1, 0, 0) in component "Tapa Nebulo"
  circle A0 centre (-0.075, 24.8216) radius 2.5
  circle A1 centre (-47.3721, 4.6708) radius 3.35
  circle A2 centre (48.4749, 5.0884) radius 3.35
  circle A3 centre (-0.0751, 0.0768) radius 3.35
  line L0 (-43.5815, 43.2263) -> (-39.9963, 46.9968)
  line L1 (-39.9963, 46.9968) -> (-37.9795, 45)
  line L2 (-37.9795, 45) -> (-38, 45)
  line L3 (-38, 45) -> (-77, 5)
  line L4 (-77, 5) -> (-38, -16)
  line L5 (-38, -16) -> (38, -16)
  line L6 (38, -16) -> (77, 5)
  line L7 (77, 5) -> (38, 45)
  line L8 (38, 45) -> (40, 47)
  line L9 (40, 47) -> (43.5784, 43.2525)
  line L10 (43.5784, 43.2525) -> (48.5784, 58.2525)
  line L11 (48.5784, 58.2525) -> (-49.7939, 58.2525)
  line L12 (-49.7939, 58.2525) -> (-43.5815, 43.2263)
  line L13 (29, 6) -> (22.4613, 6)
  line L14 (22.4613, 6) -> (22.4613, 12.5581)
  line L15 (22.4613, 12.5581) -> (29, 12.5581)
  line L16 (29, 12.5581) -> (29, 6)
  constraint horizontal L13
  constraint vertical L14
  constraint horizontal L15
  constraint vertical L16
extrude "Extrude2'''''" cut sketch "Sketch2 (6)" against normal blind 2 contours L13 L14 L15 L16 bodies 21 in component "Tapa Nebulo"
sketch "Sketch3 (5)" plane through (0, 2, 0) normal (0, -1, 0) x (1, 0, 0) in component "Tapa Nebulo"
  line L0 (22.4613, 6) -> (22.4613, 12.5581)
  line L1 (22.4613, 12.5581) -> (29, 12.5581)
  line L2 (29, 12.5581) -> (29, 6)
  line L3 (29, 6) -> (22.4613, 6)
  circle A0 centre (-0.075, 24.8216) radius 2.5
  circle A1 centre (-47.3721, 4.6708) radius 3.35
  circle A2 centre (48.4749, 5.0884) radius 3.35
  circle A3 centre (-0.0751, 0.0768) radius 3.35
  line L4 (-43.5815, 43.2263) -> (-39.9963, 46.9968)
  line L5 (-39.9963, 46.9968) -> (-37.9795, 45)
  line L6 (-37.9795, 45) -> (-38, 45)
  line L7 (-38, 45) -> (-77, 5)
  line L8 (-77, 5) -> (-38, -16)
  line L9 (-38, -16) -> (38, -16)
  line L10 (38, -16) -> (77, 5)
  line L11 (77, 5) -> (38, 45)
  line L12 (38, 45) -> (40, 47)
  line L13 (40, 47) -> (43.5784, 43.2525)
  line L14 (43.5784, 43.2525) -> (48.5784, 58.2525)
  line L15 (48.5784, 58.2525) -> (-49.7939, 58.2525)
  line L16 (-49.7939, 58.2525) -> (-43.5815, 43.2263)
  line L17 (-21, 6) -> (-27.5425, 6)
  line L18 (-27.5425, 6) -> (-27.5425, 12.5733)
  line L19 (-27.5425, 12.5733) -> (-21, 12.5733)
  line L20 (-21, 12.5733) -> (-21, 6)
  constraint horizontal L17
  constraint vertical L18
  constraint horizontal L19
  constraint vertical L20
extrude "Extrude3'''''" cut sketch "Sketch3 (5)" against normal blind 2 contours L17 L18 L19 L20 bodies 21 in component "Tapa Nebulo"
sketch "Sketch3 (6)" plane through (0, 0, -18) normal (0, 0, 1) x (-1, 0, 0) in component "DigiMod"
  line L0 (-40, -48) -> (-3, -48)
  line L1 (-3, -48) -> (-3, 0)
  line L2 (-3, 0) -> (-5, 0)
  line L3 (-40, -2) -> (-40, -48)
  line L4 (-5, 0) -> (-5, -2)
  line L5 (-5, -2) -> (-40, -2)
  line L6 (-5, 0) -> (-5, -2)
  line L7 (-5, -2) -> (-40, -2)
  constraint coincident L2 L4.start
  constraint perpendicular L2 L4
  constraint coincident L3 L5.end
  constraint perpendicular L3 L5
sketch "Sketch4 (5)" plane through (0, 0, -18) normal (0, 0, 1) x (1, 0, 0) in component "DigiMod"
extrude "Extrude24" [suppressed] in component "DigiMod"
sketch "Sketch5 (3)" plane through (0, 0, 0) normal (0, -1, 0) x (1, 0, 0) in component "DigiMod"
  line L0 (75, 0) -> (120, 0)
  line L1 (120, 0) -> (120, 2)
  line L2 (120, 2) -> (75, 2)
  line L3 (75, 0) -> (75, 2)
  line L4 (75, 2) -> (40, -18)
  line L5 (40, -20) -> (75, 0)
  line L6 (75, 2) -> (75, 0)
  constraint coincident L0.start L3.start
  constraint coincident L2.end L3.end
extrude "Extrude25" [suppressed] in component "DigiMod"
sketch "Sketch6 (3)" plane through (0, 0, 0) normal (0, -1, 0) x (1, 0, 0) in component "DigiMod"
  line L0 (-5, -20) -> (-5, -140)
  line L1 (-5, -140) -> (-40, -140)
  line L2 (-40, -140) -> (-60, -160)
  line L3 (-60, -160) -> (-58.5858, -161.4142)
  line L4 (-58.5858, -161.4142) -> (-39.1716, -142)
  line L5 (-39.1716, -142) -> (-3, -142)
  line L6 (-3, -142) -> (-3, -18)
  line L7 (-3, -18) -> (-5.0165, -18)
  line L8 (-5, -20) -> (-40, -20)
  line L9 (-75, 0) -> (-40, -20)
  line L10 (-75, 0) -> (-75, 2)
  line L11 (-74.7834, 2.4012) -> (-5.0165, -18)
  line L12 (-5, -20) -> (-5, -18)
  line L13 (-5, -18) -> (-5.0165, -18)
  line L14 (-5.0165, -18) -> (-5, -20)
  constraint coincident L0.start L8.start
  constraint coincident L7.end L11.end
  constraint coincident L7 L12.end
  constraint perpendicular L7 L12
extrude "Extrude26" [suppressed] in component "DigiMod"
component "DigiMod" placed x (1, 0, 0) y (0, 1, 0) z (0, 0, 1) at (0, 0, 0)
component "Tapas DigiMod (1)" placed x (1, 0, 0) y (0, 1, 0) z (0, 0, 1) at (-0.3871, -57.745, -0.1397)
component "NebuloSubmod" placed x (1, 0, 0) y (0, 1, 0) z (0, 0, 1) at (0, 0, 0)
component "Tapa Nebulo" placed x (1, 0, 0) y (0, 1, 0) z (0, 0, 1) at (0, 0, 0)
